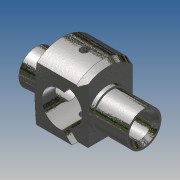
# Autodesk Inventor part: Vergasergehäuse_ra8846s
Saved by Autodesk Inventor 2021 (Build 250183000, 183)
## iProperties
Created: 2021-01-02
Part Number: Vergasergehäuse_ra8846s
Material: Stahl, galvanisiert
Document SubType Name: Modeling
Designer: Ricardo
Density: 7.85 g/cm^3
Appearance: Galvanisiert
Project: Motor
Mass: 15.0659 g
Surface Area: 20.6418 cm^2
Volume: 1.91922 cm^3
Author: Sander
Revision Number: Rev00
Autodesk Inventor part; units mm, degrees
ref_plane "YZ-Ebene" through (0, 0, 0) normal (1, 0, 0) x (0, 1, 0)
ref_plane "XZ-Ebene" through (0, 0, 0) normal (0, 1, 0) x (-1, 0, 0)
ref_plane "XY-Ebene" through (0, 0, 0) normal (0, 0, 1) x (1, 0, 0)
sketch "Skizze1" plane through (0, 0, 0) normal (0, 0, 1) x (1, 0, 0)
  line L0 (-37.19, 0) -> (27.1401, 0) projected
  line L1 (0, -2.0026) -> (0, 12.0157) projected
  line L2 (0, 3) -> (-28, 3)
  line L3 (-28, 3) -> (-28, 4.5)
  line L4 (-28, 4.5) -> (-22, 4.2)
  line L5 (0, 4.5) -> (-8.5, 4.5)
  line L6 (-8.5, 4.5) -> (-8.5, 5)
  line L7 (-8.5, 5) -> (-9.5, 5)
  line L8 (-9.5, 5) -> (-9.5, 9.2)
  line L9 (-9.5, 9.2) -> (-11, 10)
  line L10 (-11, 10) -> (-21.2825, 10)
  arc A0 (-21.2825, 10) -> (-22, 4.2) centre (17.9501, 2.2025) ccw
  line L11 (-22, 4.2) -> (17.9501, 2.2025) construction
  point P0 (0, 0)
  dimension "d14" = 6.5
  dimension "d0" = 6
  dimension "d1" = 9
  dimension "d2" = 8.4
  dimension "d3" = 1.5
  dimension "d4" = 28
  dimension "d5" = 20
  dimension "d6" = 10
  dimension "d7" = 8.5
  dimension "d8" = 22
  dimension "d9" = 1.5
  dimension "d10" = 9.5
  dimension "d11" = 40
  dimension "d12" = 0.8
  constraints: 20 end point, 4 perpendicular, 2 horizontal, 2 point on circle, 2 point on line, 1 centre point, 1 collinear, 1 parallel
  measures "d0" diameter of L2 L0
  measures "d1" diameter of L5 L0
  measures "d2" diameter of L4.end L0
  measures "d3" distance of L2.end L3.end
  measures "d4" distance from line of L1 L3.end
  measures "d5" diameter of L10 L0
  measures "d6" diameter of L7 L0
  measures "d7" distance from line of L1 L6.end
  measures "d8" distance from line of L1 L4.end
  measures "d9" horizontal distance of L8.end L9.end
  measures "d10" distance from line of L1 L8.end
  measures "d11" radius of A0
  measures "d12" vertical distance of L10.end L8.end
revolve "Umdrehung1" add sketch "Skizze1" angle 360 about axis through (-10, 0, 0) along (1, 0, 0)
sketch "Skizze2" plane through (0, 0, 0) normal (1, 0, 0) x (0, 0, -1)
  circle A0 centre (0, 0) radius 4.5 projected
  line L0 (6.5, -6.5) -> (-13.5, -6.5)
  line L1 (-13.5, -6.5) -> (-13.5, 6.5)
  line L2 (-13.5, 6.5) -> (6.5, 6.5)
  line L3 (6.5, 6.5) -> (6.5, -6.5)
  dimension "d14" = 6.5
  dimension "d15" = 6.5
  dimension "d16" = 20
  dimension "d17" = 13
  constraints: 8 end point, 2 parallel, 1 horizontal, 1 perpendicular
  measures "d14" distance from line of L3 A0.centre
  measures "d15" distance from line of L0 A0.centre
  measures "d16" distance of L1.end L2.end
  measures "d17" distance of L0.end L1.end
extrude "Extrusion1" cut sketch "Skizze2" against normal through all contours A0 | L0 L1 L2 L3 keep common part
sketch "Skizze3" plane through (-21.4344, 6.5, -6.5) normal (0, 1, 0) x (1, 0, 0)
  line L0 (11.9344, -13.0108) -> (11.9344, 0) projected
  line L1 (11.9344, 0) -> (0, 0) projected
  point P0 (21.4344, -6.5)
  point P1 (5.9344, -6.5)
  dimension "d23" = 6
  dimension "d24" = 6.5
  measures "d23" distance from line of L0 point (5.934, -6.5)
  measures "d24" distance from line of L1 point (5.934, -6.5)
hole "Bohrung1" at (-15.5, 6.5, 0) direction (0, -1, 0) diameter 9 end through all counterbore diameter 11 counterbore depth 1
sketch "Skizze4" plane through (-21.4344, -6.5, -6.5) normal (0, -1, 0) x (1, 0, 0)
  circle A0 centre (5.9344, 6.5) radius 4.5 projected
  circle A1 centre (13.9344, 6.5) radius 8
  point P0 (21.4344, 6.5)
  dimension "d32" = 16
  constraints: 2 horizontal alignment, 2 other
extrude "Extrusion2" cut sketch "Skizze4" against normal blind 1.5 contours A0 A1 | A0 A1 picked at (7.469, 6.5) picked at (18.0285, 5.8823)
ref_plane "Arbeitsebene1" through (-16.1413, 0, 10) normal (0, 0, -1) x (-1, 0, 0)
sketch "Skizze5" plane through (-16.1413, 0, 10) normal (0, 0, -1) x (-1, 0, 0)
  line L0 (-5.1413, 6.5) -> (-5.1413, -6.5) projected
  line L1 (5.1413, 6.5) -> (-5.1413, 6.5) projected
  point P0 (-16.1413, 0)
  point P1 (-0.6413, 0)
  dimension "d35" = 4.5
  dimension "d36" = 6.5
  measures "d35" distance from line of L0 point (-0.641, 0)
  measures "d36" distance from line of L1 point (-0.641, 0)
hole "Bohrung2" at (-15.5, 0, 10) direction (0, 0, -1) diameter 2 depth 16.5
sketch "Skizze7" plane through (0, 0, 0) normal (0, 1, 0) x (-1, 0, 0)
  line L0 (33.6, 0) -> (-5.6, 0) projected
  arc A0 (22, 4.2) -> (21.2825, 10) centre (-17.9501, 2.2025) ccw projected
  line L1 (21.6692, 7.7402) -> (22.6333, 0)
  point P0 (0, 0)
  dimension "d44" = 7.8
  dimension "d45" = 22.6333
  constraints: 2 end point, 1 point on line, 1 tangent
  measures "d44" distance of L1.start L1.end
  measures "d45" distance of point (0, 0) L1.end
ref_plane "Arbeitsebene2" through (-21.6692, 0, 7.7402) normal (-0.9923, 0, 0.1236) x (-0.1236, 0, -0.9923)
sketch "Skizze8" plane through (-21.6692, 0, 7.7402) normal (-0.9923, 0, 0.1236) x (-0.1236, 0, -0.9923)
  point P0 (5.0027, 0)
  point P1 (0, 0)
  point P2 (0, 0)
  constraints: 1 coincident
hole "Bohrung3" at (-21.6692, 0, 7.7402) direction (0.9923, 0, -0.1236) diameter 1.7294 depth 9.4 tip angle 118 thread size "M2x0.25" class "6H" standard "ISO Metric profile"
ref_plane "Arbeitsebene3" through (-10, 0, 0) normal (0, 0.7071, 0.7071) x (1, 0, 0)
sketch "Skizze9" plane through (-10, 0, 0) normal (0, 0.7071, 0.7071) x (1, 0, 0)
  line L0 (-27.19, 0) -> (37.1401, 0) projected
  arc A0 (-11.4344, 9.1924) -> (-12, 4.2) centre (27.9501, 2.2025) ccw projected
  line L1 (-11.7972, 6.8156) -> (-12.4054, 0) construction
  line L2 (-11.4344, 9.1924) -> (-38.4344, 9.1924)
  line L3 (0.5, 9.1924) -> (-11.4344, 9.1924) projected
  line L4 (-38.4344, 9.1924) -> (-11.7972, 6.8156)
  point P0 (10, 0)
  dimension "d54" = 27
  dimension "d69" = 26.6372
  constraints: 6 end point, 1 collinear, 1 horizontal, 1 perpendicular, 1 point on line, 1 tangent
  measures "d54" distance of L2.start L2.end
  measures "d69" horizontal distance of L2.end L1.start
ref_plane "Arbeitsebene4" through (-21.7972, 4.8193, -4.8193) normal (0.996, -0.0628, 0.0628) x (0.063, 0.998, 0)
sketch "Skizze10" plane through (-21.7972, 4.8193, -4.8193) normal (0.996, -0.0628, 0.0628) x (0.063, 0.998, 0)
  point P0 (-3.4372, 3.4236)
  point P1 (0, 0)
  point P2 (0, 0)
  constraints: 1 coincident
hole "Bohrung4" at (-21.7972, 4.8193, -4.8193) direction (0.996, -0.0628, 0.0628) diameter 1.7294 depth 7.4 tip angle 118 thread size "M2x0.25" class "6H" standard "ISO Metric profile"
chamfer "Fase1" distance 1 angle 45 1 edges at (0, -3, 0) measured on face at (0, 3.9564, -0.359)
chamfer "Fase2" distance 1 angle 45 1 edges at (-28, -3, 0) measured on face at (-28, 3.9274, -0.5983)
